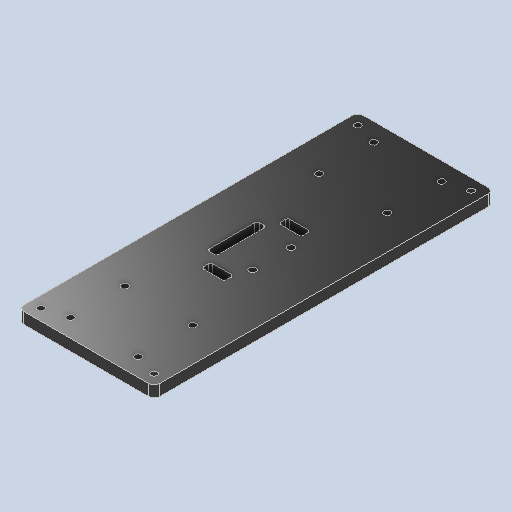
# Autodesk Inventor part: DeDuoi
Saved by Autodesk Inventor 2023 (Build 270158000, 158)
## iProperties
Created: 2023-10-13
Part Number: DeDuoi
Material: Generic
Document SubType Name: Modeling
Designer: Admins
Density: 1 g/cm^3
Appearance: Glossy - Black
Author: Admins
Autodesk Inventor part; units mm, degrees
ref_plane "YZ Plane" through (0, 0, 0) normal (1, 0, 0) x (0, 1, 0)
ref_plane "XZ Plane" through (0, 0, 0) normal (0, 1, 0) x (-1, 0, 0)
ref_plane "XY Plane" through (0, 0, 0) normal (0, 0, 1) x (1, 0, 0)
sketch "Sketch1" plane through (0, 0, 0) normal (0, 1, 0) x (-1, 0, 0)
  line L0 (-30, 75) -> (30, 75)
  line L1 (30, 75) -> (30, -75)
  line L2 (30, -75) -> (-30, -75)
  line L3 (-30, -75) -> (-30, 75)
  line L4 (30, 75) -> (25, 75)
  line L5 (25, 75) -> (25, 70)
  line L6 (25, 70) -> (30, 70)
  line L7 (30, 70) -> (30, 75)
  line L8 (-30, 75) -> (-25, 75)
  line L9 (-25, 75) -> (-25, 70)
  line L10 (-25, 70) -> (-30, 70)
  line L11 (-30, 70) -> (-30, 75)
  line L12 (30, -75) -> (25, -75)
  line L13 (25, -75) -> (25, -70)
  line L14 (25, -70) -> (30, -70)
  line L15 (30, -70) -> (30, -75)
  line L16 (-30, -75) -> (-25, -75)
  line L17 (-25, -75) -> (-25, -70)
  line L18 (-25, -70) -> (-30, -70)
  line L19 (-30, -70) -> (-30, -75)
  circle A0 centre (25, 70) radius 1.4
  circle A1 centre (-25, 70) radius 1.4
  circle A2 centre (25, -70) radius 1.4
  circle A3 centre (-25, -70) radius 1.4
  line L20 (0, 75) -> (13, 75)
  line L21 (0, 75) -> (-13, 75)
  line L22 (-9.515, 11.025) -> (9.515, 11.025)
  line L23 (9.515, 11.025) -> (9.515, -11.025)
  line L24 (9.515, -11.025) -> (-9.515, -11.025)
  line L25 (-9.515, -11.025) -> (-9.515, 11.025)
  line L26 (-9.515, 11.025) -> (9.515, -11.025) construction
  line L27 (9.515, 11.025) -> (-9.515, -11.025) construction
  line L28 (-9.515, -11.025) -> (-7.015, -11.025)
  line L29 (-7.015, -11.025) -> (-7.015, -8.525)
  line L30 (-7.015, -8.525) -> (-9.515, -8.525)
  line L31 (-9.515, -8.525) -> (-9.515, -11.025)
  line L32 (-9.515, 11.025) -> (-7.015, 11.025)
  line L33 (-7.015, 11.025) -> (-7.015, 8.525)
  line L34 (-7.015, 8.525) -> (-9.515, 8.525)
  line L35 (-9.515, 8.525) -> (-9.515, 11.025)
  circle A4 centre (-7.015, 8.525) radius 1.5
  circle A5 centre (-7.015, -8.525) radius 1.5
  line L36 (9.515, 0) -> (8.515, 0)
  line L37 (6.515, -11.025) -> (10.515, -11.025)
  line L38 (10.515, -11.025) -> (10.515, 11.025)
  line L39 (10.515, 11.025) -> (6.515, 11.025)
  line L40 (6.515, 11.025) -> (6.515, -11.025)
  line L41 (6.515, -11.025) -> (10.515, 11.025) construction
  line L42 (10.515, -11.025) -> (6.515, 11.025) construction
  line L43 (0, -75) -> (-20, -75)
  line L44 (-20, -75) -> (-20, -35)
  line L45 (-20, -35) -> (0, -35)
  line L46 (0, -35) -> (0, -75)
  line L47 (0, -75) -> (20, -75)
  line L48 (20, -75) -> (20, -35)
  line L49 (20, -35) -> (0, -35)
  line L50 (0, -35) -> (0, -75)
  line L51 (0, 75) -> (-20, 75)
  line L52 (-20, 75) -> (-20, 35)
  line L53 (-20, 35) -> (0, 35)
  line L54 (0, 35) -> (0, 75)
  line L55 (0, 35) -> (20, 35)
  line L56 (20, 35) -> (20, 75)
  line L57 (20, 75) -> (0, 75)
  line L58 (0, 75) -> (0, 35)
  line L59 (-20, -35) -> (20, -35)
  line L60 (20, -35) -> (20, -43)
  line L61 (20, -43) -> (-20, -43)
  line L62 (-20, -43) -> (-20, -35)
  line L63 (-20, 35) -> (20, 35)
  line L64 (20, 35) -> (20, 43)
  line L65 (20, 43) -> (-20, 43)
  line L66 (-20, 43) -> (-20, 35)
  line L67 (-20, 43) -> (-15, 43)
  line L68 (-15, 43) -> (15, 43)
  line L69 (15, 43) -> (15, 67)
  line L70 (15, 67) -> (-15, 67)
  line L71 (-15, 67) -> (-15, 43)
  line L72 (0, -43) -> (-15, -43)
  line L73 (15, -43) -> (15, -67)
  line L74 (15, -67) -> (-15, -67)
  line L75 (-15, -67) -> (-15, -43)
  circle A6 centre (-15, -67) radius 1.5
  circle A7 centre (15, -67) radius 1.5
  circle A8 centre (-15, -43) radius 1.5
  circle A9 centre (15, -43) radius 1.5
  circle A10 centre (-15, 67) radius 1.5
  circle A11 centre (-15, 43) radius 1.5
  circle A12 centre (15, 43) radius 1.5
  circle A13 centre (15, 67) radius 1.5
  line L76 (-20, 35) -> (20, 35)
  line L77 (20, 35) -> (20, 19)
  line L78 (20, 19) -> (-20, 19)
  line L79 (-20, 19) -> (-20, 35)
  line L80 (20, -35) -> (-20, -35)
  line L81 (-20, -35) -> (-20, -19)
  line L82 (-20, -19) -> (20, -19)
  line L83 (20, -19) -> (20, -35)
  line L84 (0, 19) -> (5, 19)
  line L85 (5, 19) -> (5, 15)
  line L86 (5, 15) -> (0, 15)
  line L87 (0, 15) -> (0, 19)
  line L88 (0, 19) -> (-5, 19)
  line L89 (-5, 19) -> (-5, 15)
  line L90 (-5, 15) -> (0, 15)
  line L91 (0, 15) -> (0, 19)
  line L92 (0, -19) -> (5, -19)
  line L93 (5, -19) -> (5, -15)
  line L94 (5, -15) -> (0, -15)
  line L95 (0, -15) -> (0, -19)
  line L96 (0, -15) -> (-5, -15)
  line L97 (-5, -15) -> (-5, -19)
  line L98 (-5, -19) -> (0, -19)
  line L99 (0, -19) -> (0, -15)
  point P0 (0, 0)
  point P1 (6.515, 11.025)
  point P2 (6.515, -11.025)
  point P3 (-5, 19)
  point P4 (5, 19)
  point P5 (0, 15)
  dimension "d0" = 60
  dimension "d1" = 150
  dimension "d2" = 5
  dimension "d3" = 5
  dimension "d4" = 5
  dimension "d5" = 5
  dimension "d6" = 5
  dimension "d7" = 5
  dimension "d8" = 5
  dimension "d9" = 5
  dimension "d10" = 2.8
  dimension "d11" = 2.8
  dimension "d39" = 19.03
  dimension "d40" = 22.05
  dimension "d41" = 2.5
  dimension "d42" = 2.5
  dimension "d43" = 2.5
  dimension "d44" = 2.5
  dimension "d45" = 3
  dimension "d46" = 3
  dimension "d47" = 1
  dimension "d48" = 4
  dimension "d54" = 20
  dimension "d55" = 40
  dimension "d56" = 20
  dimension "d57" = 20
  dimension "d58" = 40
  dimension "d59" = 20
  dimension "d60" = 8
  dimension "d61" = 8
  dimension "d62" = 5
  dimension "d63" = 30
  dimension "d64" = 24
  dimension "d65" = 24
  dimension "d66" = 3
  dimension "d67" = 3
  dimension "d68" = 3
  dimension "d69" = 3
  dimension "d70" = 3
  dimension "d71" = 3
  dimension "d72" = 3
  dimension "d75" = 16
  dimension "d76" = 16
  dimension "d77" = 5
  dimension "d78" = 4
  dimension "d79" = 5
  dimension "d80" = 5
  dimension "d81" = 4
  dimension "d82" = 5
  constraints: 200 end point, 42 parallel, 26 perpendicular, 24 horizontal, 15 point on line, 14 centre point, 14 coincident, 10 midpoint
  measures "d0" distance of L1.end L2.end
  measures "d1" distance of L0.end L1.end
  measures "d2" distance of L6.end L5.end
  measures "d3" distance of L5.end L4.end
  measures "d4" distance of L9.end L10.end
  measures "d5" distance of L8.end L9.end
  measures "d6" distance of L13.end L14.end
  measures "d7" distance of L12.end L13.end
  measures "d8" distance of L18.end L17.end
  measures "d9" distance of L17.end L16.end
  measures "d10" diameter of A0
  measures "d11" diameter of A1
  measures "d39" distance of L23.end L24.end
  measures "d40" distance of L22.end L23.end
  measures "d41" distance of L30.end L29.end
  measures "d42" distance of L29.end L28.end
  measures "d43" distance of L33.end L34.end
  measures "d44" distance of L32.end L33.end
  measures "d45" diameter of A4
  measures "d46" diameter of A5
  measures "d47" distance of L36.start L36.end
  measures "d48" distance of L39.end L38.end
  measures "d54" distance of L44.end L45.end
  measures "d55" distance of L43.end L44.end
  measures "d56" distance of L49.end L48.end
  measures "d57" distance of L53.end L52.end
  measures "d58" distance of L52.end L51.end
  measures "d59" distance of L57.end L56.end
  measures "d60" distance of L59.end L60.end
  measures "d61" distance of L64.end L63.end
  measures "d62" distance of L65.end L67.end
  measures "d63" distance of L67.end L68.end
  measures "d64" distance of L68.end L69.end
  measures "d65" distance of L73.start L73.end
  measures "d66" diameter of A6
  measures "d67" diameter of A7
  measures "d68" diameter of A8
  measures "d69" diameter of A10
  measures "d70" diameter of A11
  measures "d71" diameter of A12
  measures "d72" diameter of A13
  measures "d75" distance of L76.end L77.end
  measures "d76" distance of L80.end L81.end
  measures "d77" distance of L85.end L86.end
  measures "d78" distance of L84.end L85.end
  measures "d79" distance of L90.end L89.end
  measures "d80" distance of L94.end L93.end
  measures "d81" distance of L93.end L92.end
  measures "d82" distance of L98.end L97.end
extrude "Extrusion1" add sketch "Sketch1" along normal blind 5 contours L0 L9 A1 L10 L3 | L0 L52 L79 L78 L89 L90 L86 L85 L77 L56 L5 A0 L6 L1 L14 A2 L13 L2 L48 L83 L82 L93 L94 L96 L97 L81 L44 L17 A3 L18 L3 L10 A1 L9 | L0 L54 L70 A10 L71 A11 L65 L52 | L18 A3 L17 L2 L3 | L65 A11 L54 L53 L52 | L0 L56 L65 A12 L69 A13 L70 L54 | L53 L55 L77 L78 L79 | A11 L71 L65 | L65 A11 | L70 A13 L69 A12 L65 L54 | L54 L65 A11 L71 A10 L70 | L54 L65 A12 L56 L55 | L71 A11 L65 | L44 L61 A8 L75 A6 L74 L46 L2 | A13 L69 L70 | L70 L69 A13 | A10 L71 L70 | L70 L71 A10 | L46 L74 A7 L73 A9 L61 L48 L2 | L44 L45 L46 L61 A8 | L0 L1 L6 A0 L5 | A12 L69 L65 | L65 A12 | L74 A6 L75 A8 L61 L46 | L46 L61 A9 L73 A7 L74 | L81 L82 L83 L49 L45 | A8 L61 | L61 L75 A8 | L65 L69 A12 | L13 A2 L14 L1 L2 | L61 A9 L46 L49 L48 | A7 L73 L74 | L74 L73 A7 | A6 L75 L74 | L74 L75 A6 | L61 A8 L75 | A9 L73 L61 | L61 A9 | L61 L73 A9 | L22 L33 A4 L34 L25 | L22 L40 L24 L29 A5 L30 L25 L34 A4 L33 | L30 A5 L29 L24 L25
fillet "Fillet1" radius 2.5 4 edges at (-30, 2.5, 75) (-30, 2.5, -75) (30, 2.5, -75) (30, 2.5, 75)
fillet "Fillet2" radius 1 2 edges at (-6.515, 2.5, 11.025) (-10.515, 2.5, 11.025)
fillet "Fillet3" radius 1 2 edges at (-6.515, 2.5, -11.025) (-10.515, 2.5, -11.025)
extrude "Extrusion2" cut sketch "Sketch1" along normal blind 5 contours A11 L71 L65 | L65 A11 | L71 A11 L65 | A13 L69 L70 | L70 L69 A13 | A10 L71 L70 | L70 L71 A10 | A12 L69 L65 | L65 A12 | A8 L61 | L61 L75 A8 | L65 L69 A12 | A7 L73 L74 | L74 L73 A7 | A6 L75 L74 | L74 L75 A6 | L61 A8 L75 | A9 L73 L61 | L61 A9 | L61 L73 A9
fillet "Fillet4" radius 1 8 edges at (-5, 2.5, -15) (5, 2.5, -15) (5, 2.5, -19) (-5, 2.5, -19) (-5, 2.5, 19) (5, 2.5, 19) (5, 2.5, 15) (-5, 2.5, 15)
body "Solid1"
